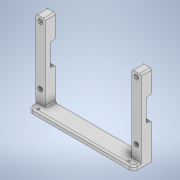
# Autodesk Inventor part: SuporteTelaLed
Saved by Autodesk Inventor 2020 (Build 240168000, 168)
## iProperties
Created: 2019-09-20
Part Number: SuporteTelaLed
Material: Generic
Document SubType Name: Modeling
Designer: Acer
Density: 1 g/cm^3
Appearance: Default
Author: Acer
Autodesk Inventor part; units mm, degrees
ref_plane "YZ Plane" through (0, 0, 0) normal (1, 0, 0) x (0, 1, 0)
ref_plane "XZ Plane" through (0, 0, 0) normal (0, 1, 0) x (-1, 0, 0)
ref_plane "XY Plane" through (0, 0, 0) normal (0, 0, 1) x (1, 0, 0)
sketch "Sketch1" plane through (0, 0, 0) normal (0, 0, 1) x (1, 0, 0)
  line L0 (-69.75, 44.75) -> (-57.75, 44.75)
  line L1 (-57.75, 44.75) -> (-57.75, -44.75)
  line L2 (-57.75, -44.75) -> (-69.75, -44.75)
  line L3 (-69.75, -44.75) -> (-69.75, 44.75)
  line L4 (57.75, 44.75) -> (69.75, 44.75)
  line L5 (69.75, 44.75) -> (69.75, -44.75)
  line L6 (69.75, -44.75) -> (57.75, -44.75)
  line L7 (57.75, -44.75) -> (57.75, 44.75)
  circle A0 centre (-63.75, 38.75) radius 1.5
  circle A1 centre (63.75, 38.75) radius 1.5
  circle A2 centre (-63.75, -38.75) radius 1.5
  circle A3 centre (63.75, -38.75) radius 1.5
  point P0 (0, 0)
  dimension "d0" = 12
  dimension "d1" = 89.5
  dimension "d2" = 12
  dimension "d3" = 89.5
  dimension "d4" = 3
  dimension "d5" = 3
  dimension "d6" = 3
  dimension "d7" = 3
  dimension "d8" = 6
  dimension "d9" = 6
  dimension "d10" = 6
  dimension "d11" = 6
  dimension "d12" = 6
  dimension "d13" = 6
  dimension "d14" = 6
  dimension "d15" = 6
  dimension "d16" = 127.5
  dimension "d17" = 63.75
  dimension "d18" = 44.75
  dimension "d19" = 44.75
  constraints: 16 end point, 4 centre point, 4 parallel, 2 horizontal, 2 perpendicular
  measures "d0" distance of L1.end L2.end
  measures "d1" distance of L0.end L1.end
  measures "d2" distance of L5.end L6.end
  measures "d3" distance of L4.end L5.end
  measures "d4" diameter of A0
  measures "d5" diameter of A1
  measures "d6" diameter of A2
  measures "d7" diameter of A3
  measures "d8" distance from line of L1 A0.centre
  measures "d9" distance from line of L0 A0.centre
  measures "d10" distance from line of L4 A1.centre
  measures "d11" distance from line of L7 A1.centre
  measures "d12" distance from line of L6 A3.centre
  measures "d13" distance from line of L7 A3.centre
  measures "d14" distance from line of L2 A2.centre
  measures "d15" distance from line of L1 A2.centre
  measures "d16" distance of A0.centre A1.centre
  measures "d17" horizontal distance of A1.centre point (0, 0)
  measures "d18" distance from line of L4 point (0, 0)
  measures "d19" distance from line of point (0, 0) L0
extrude "Extrusion1" add sketch "Sketch1" against normal blind 14
sketch "Sketch2" plane through (0, 0, 0) normal (0, 0, 1) x (1, 0, 0)
  line L0 (-69.75, -44.75) -> (-57.75, -44.75) projected
  line L1 (-57.75, -44.75) -> (-57.75, 44.75) projected
  line L2 (-57.75, 44.75) -> (-69.75, 44.75) projected
  line L3 (-69.75, 44.75) -> (-69.75, -44.75) projected
  circle A0 centre (-63.75, 38.75) radius 1.5 projected
  circle A1 centre (-63.75, -38.75) radius 1.5 projected
  line L4 (57.75, -44.75) -> (69.75, -44.75) projected
  line L5 (69.75, -44.75) -> (69.75, 44.75) projected
  line L6 (69.75, 44.75) -> (57.75, 44.75) projected
  line L7 (57.75, 44.75) -> (57.75, -44.75) projected
  circle A2 centre (63.75, -38.75) radius 1.5 projected
  circle A3 centre (63.75, 38.75) radius 1.5 projected
  circle A4 centre (-63.75, 38.75) radius 1.5 projected
  line L8 (-65.381, 35.925) -> (-67.012, 38.75)
  line L9 (-67.012, 38.75) -> (-65.381, 41.575)
  line L10 (-65.381, 41.575) -> (-62.119, 41.575)
  line L11 (-62.119, 41.575) -> (-60.488, 38.75)
  line L12 (-60.488, 38.75) -> (-62.119, 35.925)
  line L13 (-62.119, 35.925) -> (-65.381, 35.925)
  circle A5 centre (63.75, 38.75) radius 1.5 projected
  line L14 (62.119, 35.925) -> (60.488, 38.75)
  line L15 (60.488, 38.75) -> (62.119, 41.575)
  line L16 (62.119, 41.575) -> (65.381, 41.575)
  line L17 (65.381, 41.575) -> (67.012, 38.75)
  line L18 (67.012, 38.75) -> (65.381, 35.925)
  line L19 (65.381, 35.925) -> (62.119, 35.925)
  circle A6 centre (63.75, -38.75) radius 1.5 projected
  line L20 (60.488, -38.75) -> (62.119, -35.925)
  line L21 (62.119, -35.925) -> (65.381, -35.925)
  line L22 (65.381, -35.925) -> (67.012, -38.75)
  line L23 (67.012, -38.75) -> (65.381, -41.575)
  line L24 (65.381, -41.575) -> (62.119, -41.575)
  line L25 (62.119, -41.575) -> (60.488, -38.75)
  line L26 (-65.381, -41.575) -> (-67.012, -38.75)
  line L27 (-67.012, -38.75) -> (-65.381, -35.925)
  line L28 (-65.381, -35.925) -> (-62.119, -35.925)
  line L29 (-62.119, -35.925) -> (-60.488, -38.75)
  line L30 (-60.488, -38.75) -> (-62.119, -41.575)
  line L31 (-62.119, -41.575) -> (-65.381, -41.575)
  point P0 (0, 0)
  dimension "d22" = 2.825
  dimension "d23" = 2.825
  dimension "d24" = 2.825
  dimension "d25" = 2.825
  constraints: 48 end point, 4 coincident, 4 horizontal, 52 other
  measures "d22" distance from line of A0.centre L13
  measures "d23" distance from line of A3.centre L19
  measures "d24" distance from line of A2.centre L24
  measures "d25" distance from line of A1.centre L31
extrude "Extrusion2" cut sketch "Sketch2" against normal blind 6 contours L8 L9 L10 L11 L12 L13 | L14 L15 L16 L17 L18 L19 | L20 L21 L22 L23 L24 L25 | L26 L27 L28 L29 L30 L31
sketch "Sketch3" plane through (0, 0, -14) normal (0, 0, -1) x (-1, 0, 0)
  line L0 (-69.75, -44.75) -> (-57.75, -44.75) projected
  line L1 (-57.75, -44.75) -> (-57.75, 44.75) projected
  line L2 (-57.75, 44.75) -> (-69.75, 44.75) projected
  line L3 (-69.75, 44.75) -> (-69.75, -44.75) projected
  circle A0 centre (-63.75, -38.75) radius 1.5 projected
  circle A1 centre (-63.75, 38.75) radius 1.5 projected
  line L4 (57.75, -44.75) -> (69.75, -44.75) projected
  line L5 (69.75, -44.75) -> (69.75, 44.75) projected
  line L6 (69.75, 44.75) -> (57.75, 44.75) projected
  line L7 (57.75, 44.75) -> (57.75, -44.75) projected
  circle A2 centre (63.75, 38.75) radius 1.5 projected
  circle A3 centre (63.75, -38.75) radius 1.5 projected
  line L8 (-69.75, 44.75) -> (-69.75, -44.75) projected
  line L9 (-57.75, -44.75) -> (-57.75, 44.75) projected
  line L10 (-69.75, 15) -> (-57.75, 15)
  line L11 (-57.75, 15) -> (-57.75, -15)
  line L12 (-57.75, -15) -> (-69.75, -15)
  line L13 (-69.75, -15) -> (-69.75, 15)
  line L14 (57.75, -44.75) -> (57.75, 44.75) projected
  line L15 (69.75, -44.75) -> (69.75, 44.75) projected
  line L16 (57.75, 15) -> (69.75, 15)
  line L17 (69.75, 15) -> (69.75, -15)
  line L18 (69.75, -15) -> (57.75, -15)
  line L19 (57.75, -15) -> (57.75, 15)
  point P0 (0, 0)
  dimension "d28" = 30
  dimension "d29" = 15
  dimension "d30" = 15
  dimension "d31" = 30
  constraints: 16 end point, 4 parallel, 4 point on line, 2 horizontal, 2 perpendicular
  measures "d28" distance between parallel lines of L12 L10
  measures "d29" distance from line of point (0, 0) L10
  measures "d30" distance from line of point (0, 0) L16
  measures "d31" distance between parallel lines of L18 L16
extrude "Extrusion3" cut sketch "Sketch3" against normal blind 7 contours L3 L10 L1 L12 | L7 L16 L5 L18
fillet "Fillet1" radius 2 12 edges at (-63.75, 15, -14) (-63.75, 15, -7) (-63.75, -15, -14) (-63.75, -15, -7) (63.75, -15, -14) (63.75, -15, -7) (63.75, 15, -7) (63.75, 15, -14) (69.75, 44.75, -7) (57.75, 44.75, -7) (-57.75, 44.75, -7) (-69.75, 44.75, -7)
sketch "Sketch4" plane through (57.75, -44.75, 0) normal (0, -1, 0) x (1, 0, 0)
  line L0 (0, 0) -> (12, 0) projected
  line L1 (0, 0) -> (0, -14) projected
  line L2 (12, -14) -> (0, -14) projected
  line L3 (12, 0) -> (12, -14) projected
  line L4 (-127.5, 0) -> (-115.5, 0) projected
  line L5 (-127.5, 0) -> (-127.5, -14) projected
  line L6 (-115.5, -14) -> (-127.5, -14) projected
  line L7 (-115.5, 0) -> (-115.5, -14) projected
  point P0 (-57.75, 0)
extrude "Extrusion4" add sketch "Sketch4" along normal blind 12
sketch "Sketch5" plane through (57.75, -56.75, 0) normal (0, -1, 0) x (1, 0, 0)
  line L0 (12, 10) -> (-127.5, 10)
  line L1 (-127.5, 10) -> (-127.5, -14)
  line L2 (-127.5, -14) -> (12, -14)
  line L3 (12, -14) -> (12, 10)
  line L4 (12, 10) -> (-127.5, -14) construction
  line L5 (-127.5, 10) -> (12, -14) construction
  line L6 (12, -14) -> (12, 0) projected
  line L7 (12, 0) -> (0, 0) projected
  line L8 (0, 0) -> (0, -14) projected
  line L9 (0, -14) -> (12, -14) projected
  line L10 (-115.5, 0) -> (-127.5, 0) projected
  line L11 (-127.5, 0) -> (-127.5, -14) projected
  line L12 (-127.5, -14) -> (-115.5, -14) projected
  line L13 (-115.5, -14) -> (-115.5, 0) projected
  point P0 (-57.75, 0)
  point P1 (-57.75, -2)
  dimension "d37" = 139.5
  dimension "d38" = 24
  dimension "d40" = 0
  dimension "d46" = 0
  constraints: 12 end point, 2 midpoint, 2 parallel, 1 horizontal, 1 perpendicular
  measures "d37" distance of L2.end L1.end
  measures "d38" distance of L1.end L0.end
  measures "d40" distance between parallel lines of L6 L3
  measures "d46" distance between parallel lines of L2 L12
extrude "Extrusion5" add sketch "Sketch5" along normal blind 6
fillet "Fillet2" radius 5 2 edges at (69.75, -59.75, 10) (-69.75, -59.75, 10)
fillet "Fillet3" radius 2 5 edges at (0, -56.75, -14) (57.75, -56.75, -7) (69.75, -56.75, 2.5) (-69.75, -56.75, 2.5) (-57.75, -56.75, -7)
sketch "Sketch6" plane through (57.75, -62.75, 0) normal (0, -1, 0) x (1, 0, 0)
  arc A0 (-122.5, 10) -> (-127.5, 5) centre (-122.5, 5) ccw projected
  line L0 (-127.5, 5) -> (-127.5, -14) projected
  line L1 (-127.5, -14) -> (12, -14) projected
  line L2 (12, -14) -> (12, 5) projected
  arc A1 (12, 5) -> (7, 10) centre (7, 5) ccw projected
  line L3 (7, 10) -> (-122.5, 10) projected
  circle A2 centre (-117.75, 6.5) radius 1.5
  circle A3 centre (2.25, 6.5) radius 1.5
  point P0 (-57.75, 0)
  dimension "d47" = 3
  dimension "d48" = 3
  dimension "d49" = 120
  dimension "d50" = 9.75
  dimension "d51" = 3.5
  dimension "d52" = 3.5
  constraints: 2 centre point
  measures "d47" diameter of A2
  measures "d48" diameter of A3
  measures "d49" distance of A3.centre A2.centre
  measures "d50" distance from line of L0 A2.centre
  measures "d51" distance from line of L3 A2.centre
  measures "d52" distance from line of L3 A3.centre
extrude "Extrusion6" cut sketch "Sketch6" against normal up to surface (6 mm away) contours A2 | A3
sketch "Sketch7" plane through (57.75, -62.75, 0) normal (0, -1, 0) x (1, 0, 0)
  circle A0 centre (-117.75, 6.5) radius 1.5 projected
  circle A1 centre (2.25, 6.5) radius 1.5 projected
  circle A2 centre (-117.75, 6.5) radius 1.5 projected
  circle A3 centre (-117.75, 6.5) radius 2.75
  circle A4 centre (2.25, 6.5) radius 2.75
  point P0 (-57.75, 0)
  point P1 (-119.1642, 7)
  point P2 (-116.3358, 7)
  dimension "d55" = 5.5
  dimension "d56" = 5.5
  constraints: 2 centre point, 2 coincident
  measures "d55" diameter of A3
  measures "d56" diameter of A4
extrude "Extrusion7" cut sketch "Sketch7" against normal blind 2.5
equation "\"d10\" = d9"
equation "\"d11\" = d8"
equation "\"d12\" = d9"
equation "\"d13\" = d8"
equation "\"d14\" = d9"
equation "\"d15\" = d8"
equation "\"d17\" = 0.5 * d16"
equation "\"d18\" = 0.5 * d3"
equation "\"d19\" = 0.5 * d1"
equation "\"d23\" = d22"
equation "\"d24\" = d22"
equation "\"d25\" = d22"
equation "\"d29\" = 0.5 * d28"
equation "\"d30\" = d29"
equation "\"d31\" = d28"
equation "\"d52\" = d51"
body "Solid1"
